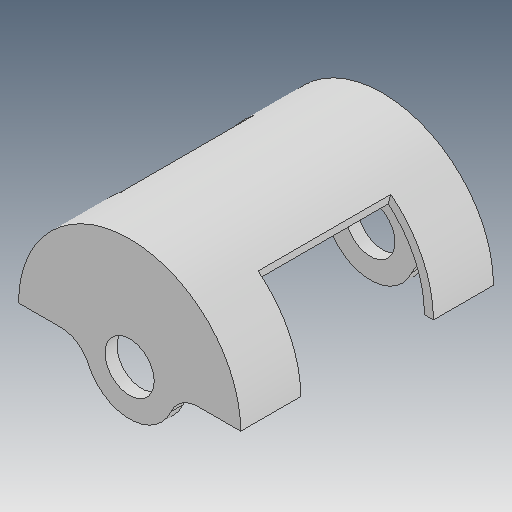
# Autodesk Inventor part: pulley_bearing_base_cover
Saved by Autodesk Inventor 2025.2 (Build 292293000, 293)
## iProperties
Created: 2025-02-16
Part Number: pulley_bearing_base_cover
Material: Generic
Document SubType Name: Modeling
Designer: email
Density: 1 g/cm^3
Appearance: Default
Author: email
Autodesk Inventor part; units mm, degrees
ref_plane "YZ Plane" through (0, 0, 0) normal (1, 0, 0) x (0, 1, 0)
ref_plane "XZ Plane" through (0, 0, 0) normal (0, 1, 0) x (-1, 0, 0)
ref_plane "XY Plane" through (0, 0, 0) normal (0, 0, 1) x (1, 0, 0)
sketch "Sketch1" plane through (0, 0, 0) normal (0, 0, 1) x (1, 0, 0)
  circle A0 centre (0, 0) radius 4.1
  circle A1 centre (0, 0) radius 17
  circle A2 centre (0, 0) radius 18.5
  line L0 (-18.5, 0) -> (18.5, 0)
  circle A3 centre (0, 0) radius 7.5
  line L1 (-7.5, 0) -> (-11.4034, 14.5675)
  line L2 (7.5, 0) -> (11.4034, 14.5675)
  point P0 (-17, 0)
  point P1 (17, 0)
  point P2 (10.978, 12.9801)
  point P3 (-10.978, 12.9801)
  dimension "d0" = 8.2
  dimension "d1" = 34
  dimension "d2" = 37
  dimension "d5" = 15
  dimension "d6" = 75
  constraints: 6 end point, 6 point on circle, 4 centre point, 4 coincident, 2 point on line, 1 equal length, 1 horizontal
  measures "d0" diameter of A0
  measures "d1" diameter of A1
  measures "d2" diameter of A2
  measures "d5" diameter of A3
  measures "d6" angle of L0 L1
extrude "Extrusion1" add sketch "Sketch1" along normal blind 19.05 contours A1 L1 A2 L2
extrude "Extrusion2" add sketch "Sketch1" against normal blind 2 contours L0 A3 A0 | A0 L0 A3 | L2 A1 L0 | A3 L1 A1 L2 | L0 A1 L1 | A1 L2 A2 L0 | A1 L1 A2 L2 | L0 A2 L1 A1
extrude "Extrusion3" add sketch "Sketch1" along normal blind 8 contours A1 L2 A2 L0 | L0 A2 L1 A1
mirror "Mirror1" about plane through (0, 15.7401, 19.05) normal (0, 0, 1)
fillet "Fillet1" radius 5 4 edges at (-7.5, 0, -1) (7.5, 0, -1) (7.5, 0, 39.1) (-7.5, 0, 39.1)
body "Solid1"
